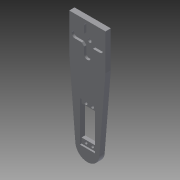
# Autodesk Inventor part: BackUpperLeg
Saved by Autodesk Inventor 2014 SP1 (Build 180222100, 222)
## iProperties
Created: 2013-09-20
Part Number: BackUpperLeg
Material: Generic
Document SubType Name: Modeling
Designer: Medrimonia
Density: 1 g/cm^3
Appearance: Default
d0: 30,000 mm
d1: 4,900 mm
d2: 10,200 mm
d3: 0,200 mm
d4: 0,200 mm
d5: 1,900 mm
d6: 0,00 deg
d7: 3,000 mm
d8: 2,000 mm
d9: 0,00 deg
d10: 5,500 mm
d11: 0,500 mm
d12: 0,00 deg
d13: 2,000 mm
d16: 2,450 mm
d17: 2,450 mm
d18: 2,000 mm
d21: 2,000 mm
d24: 2,450 mm
d25: 2,450 mm
d26: 2,450 mm
d27: 2,450 mm
d28: 2,000 mm
d31: 2,450 mm
d32: 76,150 mm
d33: 20,000 mm
d35: 0,00 deg
d36: 11,400 mm
d37: 23,500 mm
d38: 3,000 mm
d39: 2,400 mm
d40: 4,400 mm
d41: 0,500 mm
d42: 0,500 mm
d43: 60,000 mm
d44: 2,600 mm
d46: 0,00 deg
d64: 11,400 mm
d65: 23,500 mm
d68: 4,400 mm
d70: 0,500 mm
d71: 60,000 mm
d81: 0,500 mm
d92: 1,400 mm
d93: 0,00 deg
FrontUpperLegLength: 60,000 mm
FrontUpperLegKneeWidth: 20,000 mm
ServoTraceSpacing: 0,500 mm
FrontUpperLegShoulderWidth: 30,000 mm
LegServoThickness: 3,000 mm
d73: 11,400 mm
d74: 23,500 mm
d77: 4,400 mm
ServoArmWidth: 4,900 mm
ServoArmSpacing: 0,200 mm
ServoArmLength: 10,200 mm
ServoArmThickness: 1,900 mm
ServoArmHoleRequired: 3,000 mm
ServoArmHeadScrewTrace: 5,500 mm
ServoArmHeadScrewThickness: 0,500 mm
MinimalThickness: 2,000 mm
ServoArmInternFillet: 2,000 mm
ServoArmExternFillet: 2,450 mm
ServoCoreToFixation: 2,400 mm
ServoEdgeToFixation: 3,000 mm
ServoCoreWidth: 11,400 mm
ServoSpacing: 0,200 mm
ServoCoreLength: 23,500 mm
ServoFixationLength: 4,400 mm
ServoScrewDiameter: 2,000 mm
ServoScrewDiameterRequired: 2,600 mm
ServoHeadScrewTrace: 4,500 mm
ServoHeadScrewThickness: 2,500 mm
ServoExtendedSpacing: 1,000 mm
ServoAxisToCenter: 6,500 mm
Author: Medrimonia
Autodesk Inventor part; units mm, degrees
ref_plane "YZ Plane" through (0, 0, 0) normal (1, 0, 0) x (0, 1, 0)
ref_plane "XZ Plane" through (0, 0, 0) normal (0, 1, 0) x (-1, 0, 0)
ref_plane "XY Plane" through (0, 0, 0) normal (0, 0, 1) x (1, 0, 0)
sketch "Sketch1" plane through (0, 0, 0) normal (0, 1, 0) x (-1, 0, 0)
  line L0 (-15, -15) -> (15, -15)
  line L1 (15, -15) -> (15, 15)
  line L2 (15, 15) -> (-15, 15)
  line L3 (-15, 15) -> (-15, -15)
  line L4 (-15, -15) -> (15, 15) construction
  line L5 (15, -15) -> (-15, 15) construction
  line L6 (-2.45, -12.65) -> (2.45, -12.65) construction
  line L7 (2.45, -12.65) -> (2.45, 12.65) construction
  line L8 (2.45, 12.65) -> (-2.45, 12.65) construction
  line L9 (-2.45, 12.65) -> (-2.45, -12.65) construction
  line L10 (-2.45, -12.65) -> (2.45, 12.65) construction
  line L11 (2.45, -12.65) -> (-2.45, 12.65) construction
  line L12 (-12.65, -2.45) -> (12.65, -2.45) construction
  line L13 (12.65, -2.45) -> (12.65, 2.45) construction
  line L14 (12.65, 2.45) -> (-12.65, 2.45) construction
  line L15 (-12.65, 2.45) -> (-12.65, -2.45) construction
  line L16 (-12.65, -2.45) -> (12.65, 2.45) construction
  line L17 (12.65, -2.45) -> (-12.65, 2.45) construction
  line L18 (-12.85, -2.65) -> (12.85, -2.65)
  line L19 (12.85, -2.65) -> (12.85, 2.65)
  line L20 (12.85, 2.65) -> (-12.85, 2.65)
  line L21 (-12.85, 2.65) -> (-12.85, -2.65)
  line L22 (-12.85, -2.65) -> (12.85, 2.65) construction
  line L23 (12.85, -2.65) -> (-12.85, 2.65) construction
  line L24 (-2.65, -12.85) -> (2.65, -12.85)
  line L25 (2.65, -12.85) -> (2.65, 12.85)
  line L26 (2.65, 12.85) -> (-2.65, 12.85)
  line L27 (-2.65, 12.85) -> (-2.65, -12.85)
  line L28 (-2.65, -12.85) -> (2.65, 12.85) construction
  line L29 (2.65, -12.85) -> (-2.65, 12.85) construction
  point P0 (0, 0)
  point P1 (0, 0)
  dimension "d0" = 30
  dimension "d1" = 4.9
  dimension "d2" = 10.2
  dimension "d3" = 0.2
  dimension "d4" = 0.2
  constraints: 60 end point, 12 midpoint, 10 parallel, 10 perpendicular, 5 horizontal
  measures "d0" distance of L1.end L2.end
  measures "d1" distance of L14.end L12.start
  measures "d2" distance between parallel lines of L13 L7
  measures "d3" distance between parallel lines of L25 L7
  measures "d4" distance between parallel lines of L26 L8
extrude "Extrusion1" add sketch "Sketch1" along normal blind 1.9
sketch "Sketch2" plane through (0, 1.9, 0) normal (0, 1, 0) x (1, 0, 0)
  line L0 (15, 15) -> (-15, 15) projected
  line L1 (-15, 15) -> (-15, -15) projected
  line L2 (-15, -15) -> (15, -15) projected
  line L3 (15, -15) -> (15, 15) projected
  circle A0 centre (0, 0) radius 1.5
  dimension "d7" = 3
  constraints: 1 centre point, 1 coincident
  measures "d7" diameter of A0
extrude "Extrusion2" add sketch "Sketch2" along normal blind 2
sketch "Sketch3" plane through (0, 3.9, 0) normal (0, 1, 0) x (1, 0, 0)
  circle A0 centre (0, 0) radius 1.5 projected
  line L0 (15, 15) -> (-15, 15) projected
  line L1 (-15, 15) -> (-15, -15) projected
  line L2 (-15, -15) -> (15, -15) projected
  line L3 (15, -15) -> (15, 15) projected
  circle A1 centre (0, 0) radius 2.75
  dimension "d10" = 5.5
  constraints: 1 centre point, 1 coincident
  measures "d10" diameter of A1
extrude "Extrusion3" add sketch "Sketch3" along normal blind 0.5 contours L3 L2 L1 L0
chamfer "Chamfer1" distance 2 angle 45 1 edges at (-2.65, 0.95, -2.65)
fillet "Fillet1" radius 2.45 1 edges at (-12.85, 0.95, -2.65)
fillet "Fillet2" radius 2.45 1 edges at (-2.65, 0.95, -12.85)
chamfer "Chamfer2" distance 2 angle 45 1 edges at (2.65, 0.95, -2.65)
chamfer "Chamfer3" distance 2 angle 45 1 edges at (2.65, 0.95, 2.65)
fillet "Fillet3" radius 2.45 1 edges at (12.85, 0.95, -2.65)
fillet "Fillet4" radius 2.45 1 edges at (2.65, 0.95, -12.85)
fillet "Fillet5" radius 2.45 1 edges at (12.85, 0.95, 2.65)
fillet "Fillet6" radius 2.45 1 edges at (2.65, 0.95, 12.85)
chamfer "Chamfer4" distance 2 angle 45 1 edges at (-2.65, 0.95, 2.65)
fillet "Fillet7" radius 2.45 2 edges at (-2.65, 0.95, 12.85) (-12.85, 0.95, 2.65)
sketch "Sketch4" plane through (0, 0, 0) normal (0, -1, 0) x (1, 0, 0)
  line L0 (15, -15) -> (-15, -15) projected
  line L1 (-10.4, 2.65) -> (-4.65, 2.65) projected
  line L2 (-15, -15) -> (-10, -76.15)
  line L3 (-10, -76.15) -> (10, -76.15)
  line L4 (10, -76.15) -> (15, -15)
  line L5 (0, 0) -> (0, -92.3376) construction
  arc A0 (-10, -76.15) -> (10, -76.15) centre (0, -76.15) ccw
  dimension "d32" = 76.15
  dimension "d33" = 20
  constraints: 8 end point, 2 point on circle, 1 centre point, 1 midpoint, 1 parallel, 1 perpendicular, 1 other
  measures "d32" distance from line of L3 L5.start
  measures "d33" distance of L2.end L3.end
extrude "Extrusion4" add sketch "Sketch4" against normal up to surface (4.4 mm away)
sketch "Sketch5" plane through (0, 0, 0) normal (0, -1, 0) x (1, 0, 0)
  line L0 (-5.7, -48.25) -> (5.7, -48.25) construction
  line L1 (5.7, -48.25) -> (5.7, -71.75) construction
  line L2 (5.7, -71.75) -> (-5.7, -71.75) construction
  line L3 (-5.7, -71.75) -> (-5.7, -48.25) construction
  line L4 (0, 0) -> (0, -72.1654) construction
  line L5 (-5.7, -48.25) -> (-5.7, -43.85) construction
  line L6 (-5.7, -43.85) -> (5.7, -43.85) construction
  line L7 (5.7, -43.85) -> (5.7, -48.25) construction
  line L8 (5.7, -71.75) -> (5.7, -76.15) construction
  line L9 (5.7, -76.15) -> (-5.7, -76.15) construction
  line L10 (-5.7, -76.15) -> (-5.7, -71.75) construction
  circle A0 centre (-2.7, -45.85) radius 1.3
  circle A1 centre (2.7, -45.85) radius 1.3
  line L11 (-17.4512, -60) -> (18.2205, -60) construction
  circle A2 centre (-2.7, -74.15) radius 1.3
  circle A3 centre (2.7, -74.15) radius 1.3
  line L12 (-6.2, -47.75) -> (6.2, -47.75)
  line L13 (6.2, -47.75) -> (6.2, -72.25)
  line L14 (6.2, -72.25) -> (-6.2, -72.25)
  line L15 (-6.2, -72.25) -> (-6.2, -47.75)
  dimension "d36" = 11.4
  dimension "d37" = 23.5
  dimension "d38" = 3
  dimension "d39" = 2.4
  dimension "d40" = 4.4
  dimension "d41" = 0.5
  dimension "d42" = 0.5
  dimension "d43" = 60
  dimension "d44" = 2.6
  constraints: 32 end point, 8 parallel, 5 perpendicular, 4 centre point, 3 symmetric about line, 2 horizontal, 1 collinear, 8 other
  measures "d36" distance between parallel lines of L1 L3
  measures "d37" distance between parallel lines of L2 L0
  measures "d38" distance from line of L5 A0.centre
  measures "d39" distance from line of A3.centre L2
  measures "d40" distance between parallel lines of L0 L6
  measures "d41" distance between parallel lines of L0 L12
  measures "d42" distance between parallel lines of L1 L13
  measures "d43" distance from line of L11 L4.start
  measures "d44" diameter of A1
extrude "Extrusion5" cut sketch "Sketch5" against normal through all
sketch "Sketch6" plane through (0, 0, 0) normal (0, -1, 0) x (1, 0, 0)
  arc A0 (-10, -76.15) -> (10, -76.15) centre (0, -76.15) ccw projected
  line L0 (-5.7, -48.25) -> (5.7, -48.25) construction
  line L1 (5.7, -48.25) -> (5.7, -71.75) construction
  line L2 (5.7, -71.75) -> (-5.7, -71.75) construction
  line L3 (-5.7, -71.75) -> (-5.7, -48.25) construction
  line L4 (0, 0) -> (0, -72.5327) construction
  line L5 (-5.7, -48.25) -> (-5.7, -43.85) construction
  line L6 (-5.7, -43.85) -> (5.7, -43.85) construction
  line L7 (5.7, -43.85) -> (5.7, -48.25) construction
  line L8 (5.7, -71.75) -> (5.7, -76.15) construction
  line L9 (5.7, -76.15) -> (-5.7, -76.15) construction
  line L10 (-5.7, -76.15) -> (-5.7, -71.75) construction
  line L11 (-0.5684, -60) -> (35.1033, -60) construction
  line L12 (-6.2, -43.35) -> (6.2, -43.35)
  line L13 (6.2, -43.35) -> (6.2, -76.65)
  line L14 (6.2, -76.65) -> (-6.2, -76.65)
  line L15 (-6.2, -76.65) -> (-6.2, -43.35)
  dimension "d64" = 11.4
  dimension "d65" = 23.5
  dimension "d68" = 4.4
  dimension "d70" = 0.5
  dimension "d71" = 60
  dimension "d81" = 0.5
  constraints: 32 end point, 8 parallel, 5 perpendicular, 2 horizontal, 1 coincident, 1 collinear, 1 point on line, 5 other
  measures "d64" distance between parallel lines of L1 L3
  measures "d65" distance between parallel lines of L2 L0
  measures "d68" distance between parallel lines of L0 L6
  measures "d70" distance between parallel lines of L1 L13
  measures "d71" distance from line of L11 L4.start
  measures "d81" distance between parallel lines of L6 L12
extrude "Extrusion6" cut sketch "Sketch6" against normal blind 1.4
equation "\"d0\" = FrontUpperLegShoulderWidth"
equation "\"d1\" = ServoArmWidth"
equation "\"d2\" = ServoArmLength"
equation "\"d3\" = ServoArmSpacing"
equation "\"d4\" = ServoArmSpacing"
equation "\"d5\" = ServoArmThickness"
equation "\"d7\" = ServoArmHoleRequired"
equation "\"d8\" = MinimalThickness"
equation "\"d10\" = ServoArmHeadScrewTrace"
equation "\"d11\" = ServoArmHeadScrewThickness"
equation "\"d13\" = ServoArmInternFillet"
equation "\"d16\" = ServoArmExternFillet"
equation "\"d17\" = ServoArmExternFillet"
equation "\"d18\" = ServoArmInternFillet"
equation "\"d21\" = ServoArmInternFillet"
equation "\"d24\" = ServoArmExternFillet"
equation "\"d25\" = ServoArmExternFillet"
equation "\"d26\" = ServoArmExternFillet"
equation "\"d27\" = ServoArmExternFillet"
equation "\"d28\" = ServoArmInternFillet"
equation "\"d31\" = ServoArmExternFillet"
equation "\"d32\" = 0.5 * ServoCoreLength + FrontUpperLegLength + ServoFixationLength"
equation "\"d33\" = FrontUpperLegKneeWidth"
equation "\"d36\" = ServoCoreWidth"
equation "\"d37\" = ServoCoreLength"
equation "\"d38\" = ServoEdgeToFixation"
equation "\"d39\" = ServoCoreToFixation"
equation "\"d40\" = ServoFixationLength"
equation "\"d41\" = ServoTraceSpacing"
equation "\"d42\" = ServoTraceSpacing"
equation "\"d43\" = FrontUpperLegLength"
equation "\"d44\" = ServoScrewDiameterRequired"
equation "\"d64\" = ServoCoreWidth"
equation "\"d65\" = ServoCoreLength"
equation "\"d68\" = ServoFixationLength"
equation "\"d70\" = ServoTraceSpacing"
equation "\"d71\" = FrontUpperLegLength"
equation "\"d81\" = ServoTraceSpacing"
equation "\"d92\" = ServoArmThickness + ServoArmHeadScrewThickness + MinimalThickness - LegServoThickness"
equation "\"FrontUpperLegLength\" = 60"
equation "\"FrontUpperLegKneeWidth\" = 20"
equation "\"ServoTraceSpacing\" = 0.5"
equation "\"FrontUpperLegShoulderWidth\" = 30"
equation "\"LegServoThickness\" = 3"
equation "\"ServoArmWidth\" = 4.9"
equation "\"ServoArmLength\" = 10.2"
equation "\"ServoArmSpacing\" = 0.2"
equation "\"ServoArmThickness\" = 1.9"
equation "\"ServoArmHoleRequired\" = 3"
equation "\"MinimalThickness\" = 2"
equation "\"ServoArmHeadScrewTrace\" = 5.5"
equation "\"ServoArmHeadScrewThickness\" = 0.5"
equation "\"ServoArmInternFillet\" = 2"
equation "\"ServoArmExternFillet\" = 2.45"
equation "\"ServoCoreLength\" = 23.5"
equation "\"ServoFixationLength\" = 4.4"
equation "\"ServoCoreWidth\" = 11.4"
equation "\"ServoEdgeToFixation\" = 3"
equation "\"ServoCoreToFixation\" = 2.4"
equation "\"ServoScrewDiameterRequired\" = 2.6"
body "Solid1"
